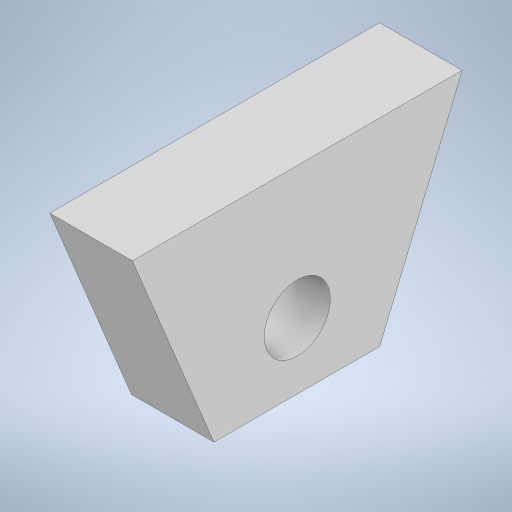
# Autodesk Inventor part: Деталь1
Saved by Autodesk Inventor 2024 (Build 280153000, 153)
## iProperties
Created: 2023-10-26
Part Number: Деталь1
Material: Типовые
Document SubType Name: Sheet Metal
Designer: Elisey
Density: 1 g/cm^3
Sheet Metal Rule: По умолчанию_мм
Appearance: По умолчанию
Author: Elisey
Autodesk Inventor part; units mm, degrees
ref_plane "YZ Plane" through (0, 0, 0) normal (1, 0, 0) x (0, 1, 0)
ref_plane "XZ Plane" through (0, 0, 0) normal (0, 1, 0) x (-1, 0, 0)
ref_plane "XY Plane" through (0, 0, 0) normal (0, 0, 1) x (1, 0, 0)
sketch "Эскиз1" plane through (0, 0, 0) normal (1, 0, 0) x (0, 1, 0)
  line L0 (0.0454, -28.3965) -> (31.0454, -28.3965)
  line L1 (0.0454, -18.2972) -> (0.0454, -38.3965)
  line L2 (24.0454, -28.3965) -> (24.0454, -48.3965)
  line L3 (24.0454, -48.3965) -> (24.0454, -8.3965)
  line L4 (24.0454, -8.3965) -> (0.0454, -18.2972)
  line L5 (0.0454, -38.3965) -> (24.0454, -48.3965)
  circle A0 centre (8.0454, -28.3965) radius 4
  point P0 (0, 0)
  point P1 (-21.9008, -17.3129)
  point P2 (7.0992, 6.6871)
  constraints: 12 end point, 3 point on line, 1 centre point, 1 perpendicular
extrude "Выдавливание1" add sketch "Эскиз1" along normal blind 10 contours A0 L0 L1 L4 L3 | L0 L2 L5 L1 A0
equation "\"Радиус_гибки\" = Толщина"
equation "\"Ширина_просечки\" = Толщина"
equation "\"Глубина_просечки\" = 0.5 * Толщина"
equation "\"Размер_просечки\" = 4 * Толщина"
equation "\"Мин_остаток\" = 2 * Толщина"
equation "\"Радиус_перехода\" = Радиус_гибки"
equation "\"Радиус_Якоби\" = Радиус_гибки"
equation "\"Размер_зазора\" = Толщина"
equation "\"Толщина\" = 0.5"
